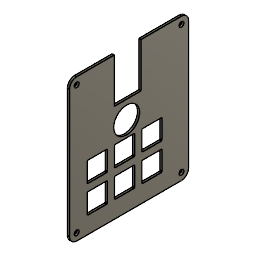
outer (Autodesk Fusion 360 design; units mm, degrees)
part number: 2025-12-20-20-24-37-630
Autodesk Fusion 360 part; units mm, degrees
sketch "plate-2025-12-20T19_09_56.435Z" plane through (0, 0, 0) normal (1, 0, 0) x (0, 1, 0)
sketch "plate-2025-12-20T19_09_56.435Z (1)" plane through (0, 0, 0) normal (1, 0, 0) x (0, 1, 0)
  line L0 (18.025, 42.475) -> (31.025, 42.475)
  line L1 (18.025, 28.475) -> (31.025, 28.475)
  line L2 (17.525, 41.975) -> (17.525, 28.975)
  line L3 (31.525, 41.975) -> (31.525, 28.975)
  arc A0 (18.025, 42.475) -> (17.525, 41.975) centre (18.025, 41.975) ccw
  arc A1 (31.525, 41.975) -> (31.025, 42.475) centre (31.025, 41.975) ccw
  arc A2 (17.525, 28.975) -> (18.025, 28.475) centre (18.025, 28.975) ccw
  arc A3 (31.025, 28.475) -> (31.525, 28.975) centre (31.025, 28.975) ccw
  line L4 (37.075, 42.475) -> (50.075, 42.475)
  line L5 (37.075, 28.475) -> (50.075, 28.475)
  line L6 (36.575, 41.975) -> (36.575, 28.975)
  line L7 (50.575, 41.975) -> (50.575, 28.975)
  arc A4 (37.075, 42.475) -> (36.575, 41.975) centre (37.075, 41.975) ccw
  arc A5 (50.575, 41.975) -> (50.075, 42.475) centre (50.075, 41.975) ccw
  arc A6 (36.575, 28.975) -> (37.075, 28.475) centre (37.075, 28.975) ccw
  arc A7 (50.075, 28.475) -> (50.575, 28.975) centre (50.075, 28.975) ccw
  line L8 (56.125, 42.475) -> (69.125, 42.475)
  line L9 (56.125, 28.475) -> (69.125, 28.475)
  line L10 (55.625, 41.975) -> (55.625, 28.975)
  line L11 (69.625, 41.975) -> (69.625, 28.975)
  arc A8 (56.125, 42.475) -> (55.625, 41.975) centre (56.125, 41.975) ccw
  arc A9 (69.625, 41.975) -> (69.125, 42.475) centre (69.125, 41.975) ccw
  arc A10 (55.625, 28.975) -> (56.125, 28.475) centre (56.125, 28.975) ccw
  arc A11 (69.125, 28.475) -> (69.625, 28.975) centre (69.125, 28.975) ccw
  line L12 (18.025, 23.425) -> (31.025, 23.425)
  line L13 (18.025, 9.425) -> (31.025, 9.425)
  line L14 (17.525, 22.925) -> (17.525, 9.925)
  line L15 (31.525, 22.925) -> (31.525, 9.925)
  arc A12 (18.025, 23.425) -> (17.525, 22.925) centre (18.025, 22.925) ccw
  arc A13 (31.525, 22.925) -> (31.025, 23.425) centre (31.025, 22.925) ccw
  arc A14 (17.525, 9.925) -> (18.025, 9.425) centre (18.025, 9.925) ccw
  arc A15 (31.025, 9.425) -> (31.525, 9.925) centre (31.025, 9.925) ccw
  line L16 (37.075, 23.425) -> (50.075, 23.425)
  line L17 (37.075, 9.425) -> (50.075, 9.425)
  line L18 (36.575, 22.925) -> (36.575, 9.925)
  line L19 (50.575, 22.925) -> (50.575, 9.925)
  arc A16 (37.075, 23.425) -> (36.575, 22.925) centre (37.075, 22.925) ccw
  arc A17 (50.575, 22.925) -> (50.075, 23.425) centre (50.075, 22.925) ccw
  arc A18 (36.575, 9.925) -> (37.075, 9.425) centre (37.075, 9.925) ccw
  arc A19 (50.075, 9.425) -> (50.575, 9.925) centre (50.075, 9.925) ccw
  line L20 (56.125, 23.425) -> (69.125, 23.425)
  line L21 (56.125, 9.425) -> (69.125, 9.425)
  line L22 (55.625, 22.925) -> (55.625, 9.925)
  line L23 (69.625, 22.925) -> (69.625, 9.925)
  arc A20 (56.125, 23.425) -> (55.625, 22.925) centre (56.125, 22.925) ccw
  arc A21 (69.625, 22.925) -> (69.125, 23.425) centre (69.125, 22.925) ccw
  arc A22 (55.625, 9.925) -> (56.125, 9.425) centre (56.125, 9.925) ccw
  arc A23 (69.125, 9.425) -> (69.625, 9.925) centre (69.125, 9.925) ccw
sketch "Sketch3" plane through (0, 0, 0) normal (1, 0, 0) x (0, 1, 0)
  line L0 (5.143, 96.836) -> (88.183, 96.836)
  line L1 (88.183, 96.836) -> (88.183, -2.424)
  line L2 (88.183, -2.424) -> (5.143, -2.424)
  line L3 (5.143, -2.424) -> (5.143, 96.836)
  line L4 (18.025, 9.425) -> (31.025, 9.425)
  line L5 (17.525, 22.925) -> (17.525, 9.925)
  line L6 (36.493, 96.836) -> (54.993, 96.836)
  line L7 (54.993, 96.836) -> (54.993, 65.836)
  line L8 (54.993, 65.836) -> (36.493, 65.836)
  line L9 (36.493, 65.836) -> (36.493, 96.836)
  circle A0 centre (10.143, 2.576) radius 1.7
  circle A1 centre (83.183, 2.576) radius 1.7
  circle A2 centre (10.143, 91.836) radius 1.7
  circle A3 centre (83.183, 91.836) radius 1.7
  circle A4 centre (44.9917, 53.2578) radius 9
  dimension "d1" = 83.04
  dimension "d2" = 99.26
  dimension "d3" = 11.849
  dimension "d4" = 12.382
  dimension "d5" = 31
  dimension "d6" = 18.5
  dimension "d7" = 31.35
  dimension "d8" = 3.4
  dimension "d9" = 3.4
  dimension "d10" = 5
  dimension "d11" = 5
  dimension "d12" = 5
  dimension "d13" = 5
  dimension "d14" = 3.4
  dimension "d15" = 3.4
  dimension "d16" = 5
  dimension "d17" = 5
  dimension "d18" = 5
  dimension "d19" = 5
  dimension "d20" = 18
  dimension "d21" = 39.8487
  constraint horizontal L0
  constraint vertical L1
  constraint horizontal L2
  constraint vertical L3
  constraint horizontal L6
  constraint vertical L7
  constraint horizontal L8
  constraint vertical L9
  constraint coincident L0 L6.start
  measures "d1" distance of L0.start L0.end
  measures "d2" distance of L0.start L2.end
  measures "d3" distance of L2 L4
  measures "d4" distance of L3 L5
  measures "d5" distance of L6.start L8.end
  measures "d6" distance of L7.end L8.end
  measures "d7" distance of L3 L9
  measures "d8" diameter of A0
  measures "d9" diameter of A1
  measures "d10" distance of L2 A0.centre
  measures "d11" distance of L3 A0.centre
  measures "d12" distance of L2 A1.centre
  measures "d13" distance of L1 A1.centre
  measures "d14" diameter of A2
  measures "d15" diameter of A3
  measures "d16" distance of L3 A2.centre
  measures "d17" distance of L0 A2.centre
  measures "d18" distance of L1 A3.centre
  measures "d19" distance of L0 A3.centre
  measures "d20" diameter of A4
  measures "d21" distance of L3 A4.centre
extrude "Extrude1" add sketch "Sketch3" along normal blind 1.5 contours L0 L1 L2 L3 L7 L8 L9
extrude "Extrude2" cut sketch "plate-2025-12-20T19_09_56.435Z (1)" along normal through all
fillet "Fillet1" radius 5 1 edges at (0.75, 88.183, 96.836)
fillet "Fillet2" radius 5 1 edges at (0.75, 5.143, 96.836)
fillet "Fillet3" radius 5 1 edges at (0.75, 5.143, -2.424)
fillet "Fillet4" radius 5 1 edges at (0.75, 88.183, -2.424)
